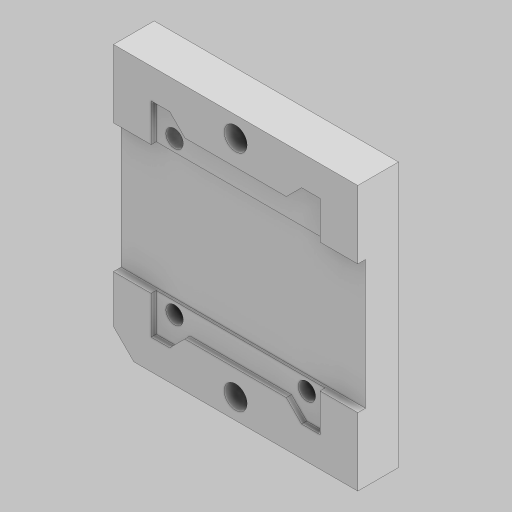
# Autodesk Inventor part: ChamberMount_c
Saved by Autodesk Inventor 2023.2 (Build 272271000, 271)
## iProperties
Created: 2023-01-17
Part Number: ChamberMount_c
Material: Generic
Document SubType Name: Modeling
Designer: splath
Density: 1 g/cm^3
Appearance: Default
Author: splath
Autodesk Inventor part; units mm, degrees
ref_plane "YZ Plane" through (0, 0, 0) normal (1, 0, 0) x (0, 1, 0)
ref_plane "XZ Plane" through (0, 0, 0) normal (0, 1, 0) x (-1, 0, 0)
ref_plane "XY Plane" through (0, 0, 0) normal (0, 0, 1) x (1, 0, 0)
sketch "Sketch1" plane through (0, 0, 0) normal (0, 0, 1) x (1, 0, 0)
  line L0 (-24, 26) -> (24, 26)
  line L1 (24, 26) -> (24, -26)
  line L2 (24, -26) -> (-24, -26)
  line L3 (-24, -26) -> (-24, 26)
  line L4 (-24, 26) -> (24, -26) construction
  line L5 (24, 26) -> (-24, -26) construction
  point P0 (0, 0)
  dimension "d2" = 48
  dimension "d3" = 52
  constraints: 12 end point, 2 midpoint, 2 parallel, 1 horizontal, 1 perpendicular
  measures "d2" distance of L1.end L2.end
  measures "d3" distance of L0.end L1.end
extrude "Extrusion1" add sketch "Sketch1" along normal blind 8
sketch "Sketch2" plane through (0, 0, 8) normal (0, 0, 1) x (1, 0, 0)
  line L0 (0, 22) -> (0, -22) construction
  point P0 (0, 0)
  point P1 (0, 0)
  dimension "d4" = 44
  constraints: 3 coincident, 2 end point, 1 midpoint, 1 vertical
  measures "d4" distance of L0.start L0.end
hole "Hole1" at (0, 22, 8) at (0, -22, 8) direction (0, 0, -1) diameter 4.5 depth 20 clearance for "Hex Head Cap Screw ISO 24017" size "M4" standard "ISO"
sketch "Sketch3" plane through (0, 0, 8) normal (0, 0, 1) x (1, 0, 0)
  line L0 (13, -20) -> (16.5, -20) projected
  line L1 (10, -17) -> (-10, -17) projected
  line L2 (13, 20) -> (16.5, 20) projected
  line L3 (-10, 17) -> (10, 17) projected
  line L4 (-13, 20) -> (-16.5, 20) projected
  line L5 (-13, 20) -> (-10, 17) projected
  line L6 (10, 17) -> (13, 20) projected
  line L7 (13, -20) -> (10, -17) projected
  line L8 (-10, -17) -> (-13, -20) projected
  line L9 (-13, -20) -> (-16.5, -20) projected
  circle A0 centre (0, 22) radius 2.25 construction
  circle A1 centre (0, -22) radius 2.25 construction
  line L10 (-24, -26) -> (24, -26) construction
  line L11 (24, -26) -> (24, 26) construction
  line L12 (24, 26) -> (-24, 26) construction
  line L13 (-24, 26) -> (-24, -26) construction
  line L14 (16.5, -20) -> (16.5, 20)
  line L15 (-16.5, 20) -> (-16.5, -20)
  point P0 (0, 0)
  constraints: 4 end point, 1 parallel, 1 perpendicular
extrude "Extrusion2" cut sketch "Sketch3" against normal blind 0.9
sketch "Sketch4" plane through (0, 0, 0) normal (0, 0, -1) x (-1, 0, 0)
  line L0 (-13, -15) -> (13, -15) construction
  line L1 (13, -15) -> (13, 15) construction
  line L2 (13, 15) -> (-13, 15) construction
  line L3 (-13, 15) -> (-13, -15) construction
  line L4 (-13, -15) -> (13, 15) construction
  line L5 (13, -15) -> (-13, 15) construction
  point P0 (0, 0)
  dimension "d16" = 26
  dimension "d17" = 30
  constraints: 12 end point, 2 midpoint, 2 parallel, 1 horizontal, 1 perpendicular
  measures "d16" distance of L2.end L1.end
  measures "d17" distance of L1.end L0.end
hole "Hole2" at (-13, 15, 0) at (-13, -15, 0) at (13, -15, 0) direction (0, 0, 1) diameter 3.4 end through all counterbore diameter 5.8 counterbore depth 3.4 clearance for "Socket Head Cap Screw ISO 4762" size "M3" standard "ISO"
chamfer "Chamfer1" distance 4 angle 45 1 edges at (-24, -26, 4)
thicken "Thicken1" operation cut thickness 0.1 both sides no extend neighbours no toward (0, 1, 0) faces at (-14.1667, 20, 7.7) (-11, 18, 7.7) (3.3333, 17, 7.4) (12, 19, 7.7) (15.3333, 20, 7.7) (11, -18, 7.7) (14.1667, -20, 7.7) (-3.3333, -17, 7.7) (-15.3333, -20, 7.7) (-12, -19, 7.7) (3.3333, 5.6667, 7.1) (16.5, -6.6667, 7.7) (-16.5, 6.6667, 7.7)
sketch "Sketch5" plane through (0, 0, 8) normal (0, 0, 1) x (1, 0, 0)
  line L0 (24, 12.65) -> (-24, 12.65)
  line L1 (-24, 12.65) -> (-24, -12.65)
  line L2 (-24, -12.65) -> (24, -12.65)
  line L3 (24, -12.65) -> (24, 12.65)
  line L4 (24, 12.65) -> (-24, -12.65) construction
  line L5 (-24, 12.65) -> (24, -12.65) construction
  line L6 (24, -26) -> (24, 26) construction
  point P0 (0, 0)
  dimension "d28" = 25.3
  constraints: 12 end point, 2 midpoint, 2 parallel, 1 collinear, 1 horizontal, 1 perpendicular
  measures "d28" distance of L2.end L0.start
extrude "Extrusion3" cut sketch "Sketch5" against normal blind 1.5
body "Solid1"
